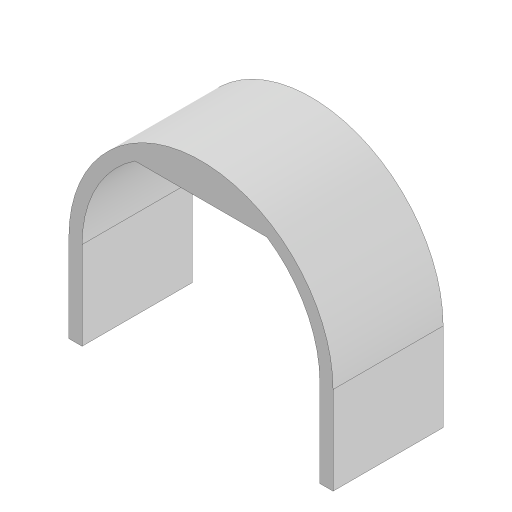
# Autodesk Inventor part: Team29_SensorHolder
Saved by Autodesk Inventor 2023 (Build 270158000, 158)
## iProperties
Created: 2023-02-17
Part Number: Team29_SensorHolder
Material: Generic
Document SubType Name: Modeling
Designer: Fariha
Density: 1 g/cm^3
Appearance: Default
Author: Fariha
Autodesk Inventor part; units mm, degrees
ref_plane "YZ Plane" through (0, 0, 0) normal (1, 0, 0) x (0, 1, 0)
ref_plane "XZ Plane" through (0, 0, 0) normal (0, 1, 0) x (-1, 0, 0)
ref_plane "XY Plane" through (0, 0, 0) normal (0, 0, 1) x (1, 0, 0)
sketch "Sketch1" plane through (0, 0, 0) normal (0, 0, 1) x (1, 0, 0)
  arc A0 (30, 0) -> (-30, 0) centre (0, 0) ccw
  line L0 (0, 0) -> (-30, 0) construction
  line L1 (0, 0) -> (30, 0) construction
  arc A1 (27, 0) -> (-27, 0) centre (0, 0) ccw
  line L2 (-15, 22.4499) -> (15, 22.4499)
  line L3 (-30, 0) -> (-27, 0)
  line L4 (27, 0) -> (30, 0)
  dimension "d0" = 30
  dimension "d1" = 180
  dimension "d2" = 3
  dimension "d3" = 30
  constraints: 10 end point, 6 point on circle, 3 collinear, 2 centre point, 2 coincident, 2 horizontal, 2 point on line
  measures "d0" radius of A0
  measures "d1" angle of L0 L1
  measures "d2" radial gap between concentric circles of A0 A1
  measures "d3" distance of L2.start L2.end
extrude "Extrusion1" add sketch "Sketch1" along normal blind 25
sketch "Sketch5" plane through (27, 0, 0) normal (0, -1, 0) x (1, 0, 0)
  line L0 (-57, 25) -> (-54, 25)
  line L1 (-54, 25) -> (-54, 0)
  line L2 (-54, 0) -> (-57, 0)
  line L3 (-57, 0) -> (-57, 25)
  line L4 (3, 0) -> (3, 25) projected
  line L5 (0, 0) -> (3, 0)
  line L6 (3, 0) -> (3, 25)
  line L7 (3, 25) -> (0, 25)
  line L8 (0, 25) -> (0, 0)
  point P0 (-27, 0)
  dimension "d6" = 3
  dimension "d7" = 25
  dimension "d8" = 3
  dimension "d9" = 25
  constraints: 16 end point, 4 parallel, 2 horizontal, 2 perpendicular
  measures "d6" distance of L1.end L2.end
  measures "d7" distance of L0.end L1.end
  measures "d8" distance of L7.end L4.end
  measures "d9" distance of L4.end L5.end
extrude "Extrusion2" add sketch "Sketch5" along normal blind 20
body "Solid1"
